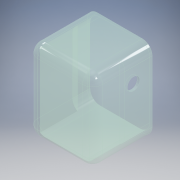
# Autodesk Inventor part: Case_Top
Saved by Autodesk Inventor 2020 (Build 240168000, 168)
## iProperties
Created: 2020-02-24
Part Number: Case_Top
Material: 일반
Document SubType Name: Modeling
Designer: Knowblesse
Density: 1 g/cm^3
Appearance: 기본값
Author: Knowblesse
## iProperties of the stored document _3D 인쇄.ipt
Created: 2020-02-24
Part Number: _3D 인쇄
Material: 일반
Document SubType Name: Modeling
Designer: Knowblesse
Density: 1 g/cm^3
Appearance: 기본값
Author: Knowblesse
Autodesk Inventor part; units mm, degrees
ref_plane "YZ Plane" through (0, 0, 0) normal (1, 0, 0) x (0, 1, 0)
ref_plane "XZ Plane" through (0, 0, 0) normal (0, 1, 0) x (-1, 0, 0)
ref_plane "XY Plane" through (0, 0, 0) normal (0, 0, 1) x (1, 0, 0)
sketch "스케치1" plane through (0, 0, 0) normal (0, 0, 1) x (1, 0, 0)
  line L0 (0, 0) -> (12, 0)
  line L1 (12, 0) -> (12, 15.4)
  line L2 (12, 15.4) -> (0, 15.4)
  line L3 (0, 15.4) -> (0, 0)
  line L4 (-0.5, 15.9) -> (12.5, 15.9)
  line L5 (12.5, 15.9) -> (12.5, -0.5)
  line L6 (12.5, -0.5) -> (-0.5, -0.5)
  line L7 (-0.5, -0.5) -> (-0.5, 15.9)
  dimension "d0" = 12
  dimension "d1" = 15.4
  dimension "d2" = 0.5
  constraints: 16 end point, 4 parallel, 2 perpendicular, 1 horizontal, 3 other
  measures "d0" distance of L1.end L2.end
  measures "d1" distance between parallel lines of L0 L2
  measures "d2" distance between parallel lines of L2 L4
extrude "돌출1" add sketch "스케치1" along normal blind 5
sketch "스케치2" plane through (0, 0, 5) normal (0, 0, 1) x (1, 0, 0)
  line L0 (-0.5, 15.9) -> (-0.5, -0.5) projected
  line L1 (-0.5, -0.5) -> (12.5, -0.5) projected
  line L2 (12.5, -0.5) -> (12.5, 15.9) projected
  line L3 (12.5, 15.9) -> (-0.5, 15.9) projected
  line L4 (12, 0) -> (0, 0) projected
  line L5 (0, 0) -> (0, 15.4) projected
  line L6 (0, 15.4) -> (12, 15.4) projected
  line L7 (12, 15.4) -> (12, 0) projected
  line L8 (1, 15.4) -> (1, 0)
  line L9 (12, 0) -> (0, 0) projected
  line L10 (11, 15.4) -> (11, 0)
  line L11 (0, 15.4) -> (12, 15.4) projected
  point P0 (11, 15.4)
  dimension "d5" = 1
  dimension "d6" = 1
  constraints: 4 end point, 4 point on line, 2 perpendicular
  measures "d5" distance between parallel lines of L5 L8
  measures "d6" distance between parallel lines of L7 L10
extrude "돌출2" add sketch "스케치2" along normal blind 6 contours L3 L2 L1 L0 | L4 L10 L6 L7 | L4 L5 L6 L8
fillet "모깎기1" radius 2 4 edges at (0, 15.4, 2.5) (12, 15.4, 2.5) (12, 0, 2.5) (0, 0, 2.5)
sketch "스케치3" plane through (0, 0, 11) normal (0, 0, 1) x (1, 0, 0)
  line L0 (-0.5, -0.5) -> (12.5, -0.5) projected
  line L1 (12.5, -0.5) -> (12.5, 15.9) projected
  line L2 (12.5, 15.9) -> (-0.5, 15.9) projected
  line L3 (-0.5, 15.9) -> (-0.5, -0.5) projected
  line L4 (10, 0) -> (2, 0) projected
  arc A0 (1, 0.2679) -> (2, 0) centre (2, 2) ccw projected
  line L5 (1, 0.2679) -> (1, 15.1321) projected
  arc A1 (2, 15.4) -> (1, 15.1321) centre (2, 13.4) ccw projected
  line L6 (2, 15.4) -> (10, 15.4) projected
  arc A2 (11, 15.1321) -> (10, 15.4) centre (10, 13.4) ccw projected
  line L7 (11, 15.1321) -> (11, 0.2679) projected
  arc A3 (10, 0) -> (11, 0.2679) centre (10, 2) ccw projected
  point P0 (0, 0)
extrude "돌출3" add sketch "스케치3" along normal blind 1 contours L3 L2 L1 L0 | L4 A0 L5 A1 L6 A2 L7 A3
sketch "스케치4" plane through (12.5, -0.5, 0) normal (1, 0, 0) x (0, 0, -1)
  line L0 (-5, 13.9) -> (-5, 2.5) projected
  line L1 (-11, 15.9) -> (0, 15.9) projected
  point P0 (0, 0.5)
  point P1 (-3.75, 11.4)
  dimension "d12" = 1.25
  dimension "d14" = 4.5
  measures "d12" distance from line of L0 point (-3.75, 11.4)
  measures "d14" distance from line of L1 point (-3.75, 11.4)
hole "구멍1" at (12.5, 10.9, 3.75) direction (-1, 0, 0) diameter 2.5 depth 0.5 tip angle 118
fillet "모깎기2" radius 2 8 edges at (12.5, -0.5, 6) (-0.5, -0.5, 6) (12.5, 15.9, 6) (-0.5, 15.9, 6) (12.5, 7.7, 12) (6, -0.5, 12) (-0.5, 7.7, 12) (6, 15.9, 12)
sketch "스케치5" plane through (0, 0, 5) normal (0, 0, -1) x (-1, 0, 0)
  arc A0 (-1, 0.2679) -> (0, 2) centre (-2, 2) ccw projected
  line L0 (0, 2) -> (0, 13.4) projected
  arc A1 (0, 13.4) -> (-1, 15.1321) centre (-2, 13.4) ccw projected
  line L1 (-1, 0.2679) -> (-1, 15.1321) projected
  point P0 (0, 0)
extrude "돌출4" add sketch "스케치5" along normal blind 1.5
